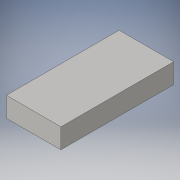
# Autodesk Inventor part: Battery Pack
Saved by Autodesk Inventor 2016 (Build 200138000, 138)
## iProperties
Created: 2016-10-06
Part Number: Battery Pack
Material: Generic
Document SubType Name: Modeling
Designer: sheehm
Density: 1 g/cm^3
Appearance: Default
Author: sheehm
Autodesk Inventor part; units mm, degrees
ref_plane "YZ Plane" through (0, 0, 0) normal (1, 0, 0) x (0, 1, 0)
ref_plane "XZ Plane" through (0, 0, 0) normal (0, 1, 0) x (-1, 0, 0)
ref_plane "XY Plane" through (0, 0, 0) normal (0, 0, 1) x (1, 0, 0)
sketch "Sketch1" plane through (0, 0, 0) normal (0, 1, 0) x (-1, 0, 0)
  line L0 (6.7307, 14.4851) -> (-26.9693, 14.4851)
  line L1 (-26.9693, 14.4851) -> (-26.9693, -55.1149)
  line L2 (-26.9693, -55.1149) -> (6.7307, -55.1149)
  line L3 (6.7307, -55.1149) -> (6.7307, 14.4851)
  point P0 (0, 0)
  dimension "d0" = 33.7
  dimension "d1" = 69.6
  constraints: 8 end point, 2 parallel, 1 horizontal, 1 perpendicular
  measures "d0" distance of L2.end L1.end
  measures "d1" distance of L1.end L0.end
extrude "Extrusion1" add sketch "Sketch1" along normal blind 12.3
body "Solid1"
